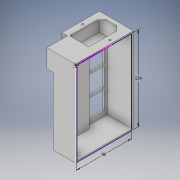
# Autodesk Inventor part: Case_Cover
Saved by Autodesk Inventor 2019 (Build 230136000, 136)
## iProperties
Created: 2019-02-06
Part Number: Case_Cover
Material: Generic
Document SubType Name: Modeling
Designer: Jorian Bruslind
Density: 1 g/cm^3
Appearance: Default
Author: Jorian Bruslind
Autodesk Inventor part; units mm, degrees
ref_plane "YZ Plane" through (0, 0, 0) normal (1, 0, 0) x (0, 1, 0)
ref_plane "XZ Plane" through (0, 0, 0) normal (0, 1, 0) x (-1, 0, 0)
ref_plane "XY Plane" through (0, 0, 0) normal (0, 0, 1) x (1, 0, 0)
sketch "Sketch1" plane through (0, 0, 0) normal (0, 1, 0) x (-1, 0, 0)
  line L0 (0, 0) -> (0, -2.1)
  line L1 (0, -2.1) -> (38.146, -2.1)
  line L2 (0, 0) -> (0, 81)
  line L3 (0, 81) -> (0, 83.1)
  line L4 (0, 83.1) -> (33, 83.1)
  line L5 (38.146, -2.1) -> (38.146, 33.9)
  line L6 (38.146, -2.1) -> (74.146, -2.1) construction
  line L7 (33, 83.1) -> (33, 33.9)
  line L8 (33, 33.9) -> (38.146, 33.9)
  dimension "d0" = 2.1
  dimension "d1" = 38.146
  dimension "d2" = 81
  dimension "d3" = 2.1
  dimension "d4" = 33
  dimension "d5" = 36
  dimension "d6" = 90
  dimension "d28" = 5.146
  constraints: 18 end point, 4 vertical, 3 horizontal, 2 perpendicular, 1 point on line
  measures "d0" distance of L0.start L0.end
  measures "d1" distance of L0.end L1.end
  measures "d2" distance of L0.start L2.end
  measures "d3" distance of L2.end L3.end
  measures "d4" distance of L3.end L4.end
  measures "d5" distance of L1.end L5.end
  measures "d6" angle of L6 L5
  measures "d28" distance of L7.end L5.end
extrude "Extrusion1" add sketch "Sketch1" along normal blind 126
sketch "Sketch2" plane through (0, 0, 83.1) normal (1, 0, 0) x (0, 0, -1)
  line L0 (54.7, 124) -> (0, 124) projected
  line L1 (0, 126) -> (0, 124)
  line L2 (0, 0) -> (0, 126) projected
  line L3 (0, 124) -> (2, 124)
  line L4 (2, 124) -> (82, 124)
  line L5 (82, 124) -> (82, 0)
  line L6 (82, 0) -> (2, 0)
  line L7 (2, 0) -> (2, 124)
  point P0 (83.1, 0)
  dimension "d10" = 2
  dimension "d11" = 2
  dimension "d12" = 80
  dimension "d13" = 124
  constraints: 12 end point, 2 parallel, 2 perpendicular, 1 horizontal, 1 point on line
  measures "d10" distance of L0.end L1.end
  measures "d11" distance of L1.end L3.end
  measures "d12" distance of L5.end L6.end
  measures "d13" distance of L4.end L5.end
sketch "Sketch3" plane through (-38.146, 0, -2.1) normal (-1, 0, 0) x (0, 0, 1)
  line L0 (0, 126) -> (36, 126) projected
  line L1 (0, 126) -> (0, 96.5)
  line L2 (0, 0) -> (0, 126) projected
  line L3 (0, 96.5) -> (6.5, 96.5)
  line L4 (6.5, 96.5) -> (33.5, 96.5)
  line L5 (33.5, 96.5) -> (33.5, 69.5)
  line L6 (33.5, 69.5) -> (6.5, 69.5)
  line L7 (6.5, 69.5) -> (6.5, 96.5)
  line L8 (6.5, 69.5) -> (6.5, 66.5)
  line L9 (6.5, 66.5) -> (33.5, 66.5)
  line L10 (33.5, 66.5) -> (33.5, 39.5)
  line L11 (33.5, 39.5) -> (6.5, 39.5)
  line L12 (6.5, 39.5) -> (6.5, 66.5)
  line L13 (6.5, 39.5) -> (6.5, 36.5)
  line L14 (6.5, 36.5) -> (33.5, 36.5)
  line L15 (33.5, 36.5) -> (33.5, 9.5)
  line L16 (33.5, 9.5) -> (6.5, 9.5)
  line L17 (6.5, 9.5) -> (6.5, 36.5)
  dimension "d32" = 29.5
  dimension "d33" = 6.5
  dimension "d34" = 27
  dimension "d35" = 27
  dimension "d36" = 3
  dimension "d37" = 27
  dimension "d38" = 27
  dimension "d39" = 3
  dimension "d40" = 27
  dimension "d41" = 27
  constraints: 32 end point, 6 parallel, 4 horizontal, 3 perpendicular, 2 vertical, 1 point on line
  measures "d32" distance of L0.start L1.end
  measures "d33" distance of L1.end L3.end
  measures "d34" distance of L5.end L6.end
  measures "d35" distance of L4.end L5.end
  measures "d36" distance of L6.end L8.end
  measures "d37" distance of L10.end L11.end
  measures "d38" distance of L9.end L10.end
  measures "d39" distance of L11.end L13.end
  measures "d40" distance of L15.end L16.end
  measures "d41" distance of L14.end L15.end
sketch "Sketch4" plane through (-33, 0, 33.9) normal (-1, 0, 0) x (0, 0, 1)
  line L0 (0, 126) -> (49.2, 126) projected
  line L1 (49.2, 126) -> (-2, 126)
  line L2 (-2, 126) -> (-2, 99)
  line L3 (-2, 99) -> (49.2, 99)
  line L4 (49.2, 99) -> (49.2, 126)
  point P0 (-33.9, 0)
  dimension "d24" = 51.2
  dimension "d25" = 27
  constraints: 8 end point, 2 parallel, 1 horizontal, 1 perpendicular
  measures "d24" distance of L3.end L2.end
  measures "d25" distance of L2.end L1.end
extrude "Extrusion2" add sketch "Sketch4" along normal blind 9
sketch "Sketch5" plane through (-38.146, 0, -2.1) normal (-1, 0, 0) x (0, 0, 1)
  line L0 (0, 0) -> (0, 126) projected
  line L1 (36, 99) -> (85.2, 99) projected
  line L2 (0, 126) -> (55, 126)
  line L3 (55, 126) -> (55, 99)
  line L4 (55, 99) -> (0, 99)
  line L5 (0, 99) -> (0, 126)
  point P0 (2.1, 0)
  point P1 (85.2, 126)
  dimension "d98" = 55
  constraints: 8 end point, 2 parallel, 1 horizontal, 1 perpendicular, 1 point on line
  measures "d98" distance of L3.end L4.end
extrude "Extrusion5" add sketch "Sketch5" along normal blind 12
shell "Shell3" thickness 2 removed faces 1 at (0, 42, 54.7)
extrude "Extrusion6" cut sketch "Sketch3" against normal blind 2
sketch "Sketch6" plane through (0, 126, 0) normal (0, 1, 0) x (1, 0, 0)
  line L0 (0, 2.1) -> (-50.146, 2.1) projected
  line L1 (0, 2.1) -> (0, -3.4)
  line L2 (0, -81.1) -> (0, 0.1) projected
  line L3 (0, 2.1) -> (5.5, 2.1) construction
  line L4 (0, -3.4) -> (-12, -3.4)
  line L5 (0, -83.1) -> (0, 2.1) projected
  line L6 (0, -3.4) -> (12, -3.4) construction
  line L7 (-12, -3.4) -> (-12, -9.9)
  line L8 (-12, -3.4) -> (-18.5, -3.4)
  line L9 (-18.5, -3.4) -> (-12, -9.9)
  line L10 (-18.5, -3.4) -> (-34.5, -3.4)
  line L11 (-34.5, -3.4) -> (-34.5, -9.9)
  line L12 (-34.5, -9.9) -> (-41, -9.9)
  line L13 (-41, -9.9) -> (-34.5, -3.4)
  line L14 (-41, -9.9) -> (-41, -48.8)
  line L15 (-41, -48.8) -> (-38.5, -48.8)
  line L16 (-12, -9.9) -> (-12, -48.8)
  line L17 (-12, -9.9) -> (26.9, -9.9) construction
  line L18 (-12, -48.8) -> (-14.5, -48.8)
  arc A0 (-14.5, -51.3) -> (-12, -48.8) centre (-14.5, -48.8) ccw
  arc A1 (-41, -48.8) -> (-38.5, -51.3) centre (-38.5, -48.8) ccw
  line L19 (-38.5, -51.3) -> (-14.5, -51.3)
  point P0 (0, 0)
  point P1 (-48.146, 2.1)
  dimension "d51" = 5.5
  dimension "d52" = 90
  dimension "d66" = 12
  dimension "d67" = 180
  dimension "d68" = 6.5
  dimension "d69" = 6.5
  dimension "d70" = 16
  dimension "d72" = 6.5
  dimension "d73" = 6.5
  dimension "d74" = 38.9
  dimension "d75" = 2.5
  dimension "d76" = 38.9
  dimension "d77" = 90
  dimension "d78" = 2.5
  dimension "d82" = 24
  constraints: 34 end point, 7 horizontal, 4 perpendicular, 4 point on circle, 3 equal length, 2 centre point, 2 coincident, 2 vertical, 1 collinear, 1 parallel
  measures "d51" distance of L0.start L1.end
  measures "d52" angle of L1 L3
  measures "d66" distance of L1.end L4.end
  measures "d67" angle of L4 L6
  measures "d68" distance of L4.end L7.end
  measures "d69" distance of L4.end L8.end
  measures "d70" distance of L8.end L10.end
  measures "d72" distance of L10.end L11.end
  measures "d73" distance of L11.end L12.end
  measures "d74" distance of L12.end L14.end
  measures "d75" distance of L14.end L15.end
  measures "d76" distance of L7.end L16.end
  measures "d77" angle of L16 L17
  measures "d78" distance of L16.end L18.end
  measures "d82" distance of L19.start L19.end
extrude "Extrusion8" cut sketch "Sketch6" against normal blind 2 contours L16 A0 L19 A1 L14 L12 L11 L10 L9 | L11 L12 L13
sketch "Sketch7" plane through (0, 126, 0) normal (0, 1, 0) x (1, 0, 0)
  line L0 (-12, -9.9) -> (-12, -48.8) projected
  line L1 (-41, -27.85) -> (-34.5, -27.85) construction
  line L2 (-14.5, -51.3) -> (-38.5, -51.3) projected
  line L3 (-34.5, -3.4) -> (-18.5, -3.4) projected
  line L4 (-18.5, -3.4) -> (-18.5, -26.9)
  line L5 (-18.5, -26.9) -> (-12, -26.9)
  line L6 (-12, -26.9) -> (-5.5, -26.9)
  circle A0 centre (-5.5, -26.9) radius 1.5
  line L7 (-18.5, -26.9) -> (-41, -26.9)
  line L8 (-18.5, -26.9) -> (4, -26.9) construction
  line L9 (-41, -26.9) -> (-45.5, -26.9)
  circle A1 centre (-45.5, -26.9) radius 1.5
  point P0 (0, 0)
  point P1 (-41, -46.9)
  point P2 (-38.146, -51.3)
  dimension "d92" = 23.5
  dimension "d93" = 6.5
  dimension "d94" = 3
  dimension "d95" = 180
  dimension "d96" = 4.5
  dimension "d97" = 3
  dimension "d99" = 23.5
  constraints: 14 end point, 3 point on line, 2 centre point, 2 coincident, 2 horizontal, 1 collinear, 1 perpendicular, 1 vertical
  measures "d92" distance of L3.end L4.end
  measures "d93" distance of L5.end L6.end
  measures "d94" diameter of A0
  measures "d95" angle of L7 L8
  measures "d96" distance of L7.end L9.end
  measures "d97" diameter of A1
  measures "d99" distance from line of L3 A1.centre
extrude "Extrusion9" cut sketch "Sketch7" against normal blind 2
sketch "Sketch8" plane through (-33, 0, 33.9) normal (-1, 0, 0) x (0, 0, 1)
  line L0 (-36, 0) -> (-36, 126) projected
  line L1 (-36, 0) -> (3.366, 0)
  line L2 (49.2, 0) -> (-36, 0) projected
  line L3 (3.366, 0) -> (3.366, 9.776)
  circle A0 centre (3.366, 9.776) radius 1.5
  line L4 (3.366, 9.776) -> (3.366, 39.776)
  line L5 (3.366, 39.776) -> (3.366, 69.776)
  circle A1 centre (3.366, 39.776) radius 1.5
  circle A2 centre (3.366, 69.776) radius 1.5
  point P0 (-33.9, 0)
  dimension "d100" = 39.366
  dimension "d101" = 9.776
  dimension "d102" = 3
  dimension "d103" = 30
  dimension "d104" = 30
  dimension "d105" = 3
  dimension "d106" = 3
  constraints: 8 end point, 3 centre point, 3 coincident, 2 point on line, 1 perpendicular, 1 vertical
  measures "d100" distance of L0.start L1.end
  measures "d101" distance of L1.end L3.end
  measures "d102" diameter of A0
  measures "d103" distance of L4.start L4.end
  measures "d104" distance of L4.end L5.end
  measures "d105" diameter of A1
  measures "d106" diameter of A2
extrude "Extrusion10" cut sketch "Sketch8" against normal blind 1.5
sketch "Sketch9" plane through (-33, 0, 33.9) normal (-1, 0, 0) x (0, 0, 1)
  line L0 (0, 0) -> (49.2, 0) projected
  line L1 (49.2, 0) -> (41.7, 0)
  line L2 (41.7, 0) -> (41.7, 10.5)
  line L3 (41.7, 10.5) -> (41.7, 15)
  circle A0 centre (41.7, 10.5) radius 1.5
  circle A1 centre (41.7, 15) radius 1.5
  point P0 (-33.9, 0)
  dimension "d109" = 7.5
  dimension "d110" = 10.5
  dimension "d111" = 4.5
  dimension "d112" = 3
  dimension "d113" = 3
  constraints: 6 end point, 2 centre point, 2 coincident, 2 point on line, 1 vertical
  measures "d109" distance of L0.end L1.end
  measures "d110" distance of L1.end L2.end
  measures "d111" distance of L2.end L3.end
  measures "d112" diameter of A0
  measures "d113" diameter of A1
extrude "Extrusion11" cut sketch "Sketch9" against normal blind 1.5
body "Solid1"
